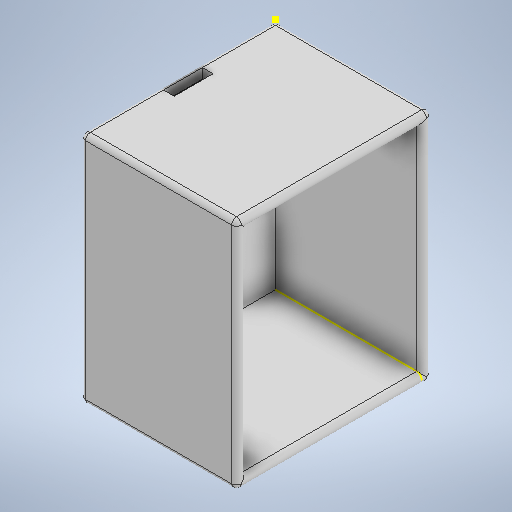
# Autodesk Inventor part: box
Saved by Autodesk Inventor 2025.2 (Build 292293000, 293)
## iProperties
Created: 2025-01-12
Part Number: box
Material: Generic
Document SubType Name: Modeling
Designer: sujay
Density: 1 g/cm^3
Appearance: Default
Author: sujay
Autodesk Inventor part; units mm, degrees
ref_plane "YZ Plane" through (0, 0, 0) normal (1, 0, 0) x (0, 1, 0)
ref_plane "XZ Plane" through (0, 0, 0) normal (0, 1, 0) x (-1, 0, 0)
ref_plane "XY Plane" through (0, 0, 0) normal (0, 0, 1) x (1, 0, 0)
sketch "Sketch1" plane through (0, 0, 0) normal (0, 0, 1) x (1, 0, 0)
  line L0 (0, 0) -> (101.6, 0)
  line L1 (101.6, 0) -> (101.6, 152.4)
  line L2 (101.6, 152.4) -> (0, 152.4)
  line L3 (0, 152.4) -> (0, 0)
  dimension "d0" = 101.6
  dimension "d1" = 152.4
  constraints: 8 end point, 2 parallel, 1 horizontal, 1 perpendicular
  measures "d0" distance of L2.end L1.end
  measures "d1" distance of L1.end L0.end
sketch "Sketch2" plane through (0, 0, 0) normal (0, 0, 1) x (1, 0, 0)
  point P0 (0, 0)
sketch "Sketch3" plane through (0, 0, 0) normal (0, 0, 1) x (1, 0, 0)
  point P0 (0, 0)
extrude "Extrusion1" add sketch "Sketch1" along normal blind 127
sketch "Sketch4" plane through (101.6, 0, 0) normal (1, 0, 0) x (0, 0, -1)
  line L0 (0, 0) -> (-127, 0) projected
  line L1 (0, 0) -> (-6.35, 0)
  line L2 (-6.35, 0) -> (-6.35, 6.35)
  line L3 (-6.35, 6.35) -> (0, 6.35)
  line L4 (0, 6.35) -> (0, 0)
  line L5 (-6.35, 6.35) -> (-120.65, 6.35)
  line L6 (-120.65, 6.35) -> (-120.65, 146.05)
  line L7 (-120.65, 146.05) -> (-6.35, 146.05)
  line L8 (-6.35, 146.05) -> (-6.35, 6.35)
  dimension "d4" = 6.35
  dimension "d5" = 6.35
  dimension "d6" = 114.3
  dimension "d7" = 139.7
  constraints: 16 end point, 4 parallel, 2 horizontal, 2 perpendicular
  measures "d4" distance of L2.end L3.end
  measures "d5" distance of L1.end L2.end
  measures "d6" distance of L6.end L7.end
  measures "d7" distance of L5.end L6.end
extrude "Extrusion2" cut sketch "Sketch4" against normal blind 95.25 contours L5 L6 L7 L8
fillet "Fillet1" radius 3.175 8 edges at (101.6, 146.05, 63.5) (101.6, 152.4, 63.5) (101.6, 76.2, 127) (101.6, 76.2, 120.65) (101.6, 76.2, 6.35) (101.6, 76.2, 0) (101.6, 6.35, 63.5) (101.6, 0, 63.5)
fillet "Fillet2" radius 3.175 8 edges at (100.6701, 151.4701, 126.0701) (49.2126, 152.4, 127) (100.6701, 151.4701, 0.9299) (49.2126, 152.4, 0) (100.6701, 0.9299, 126.0701) (49.2126, 0, 127) (100.6701, 0.9299, 0.9299) (49.2126, 0, 0)
fillet "Fillet3" radius 3.175 8 edges at (0, 0.9299, 0.9299) (0, 0, 63.5) (0, 0.9299, 126.0701) (0, 76.2, 127) (0, 151.4701, 126.0701) (0, 152.4, 63.5) (0, 151.4701, 0.9299) (0, 76.2, 0)
sketch "Sketch5" plane through (6.35, 6.35, 6.35) normal (0, 0, 1) x (1, 0, 0)
  line L0 (92.075, 0) -> (0, 0) projected
  arc A0 (95.25, -3.175) -> (92.075, 0) centre (92.075, -3.175) ccw projected
  line L1 (92.075, 0) -> (89.535, 0)
  line L2 (92.075, 0) -> (94.615, 0) construction
  line L3 (91.2996, 0) -> (88.936, -0.9299)
  point P0 (-6.35, -6.35)
  constraints: 6 end point, 2 horizontal, 1 collinear, 1 point on line
sketch "Sketch6" plane through (6.35, 6.35, 6.35) normal (0, 0, 1) x (1, 0, 0)
  point P0 (-6.35, -6.35)
sketch "Sketch7" plane through (98.425, 152.4, 123.825) normal (0, 1, 0) x (1, 0, 0)
  line L0 (-95.25, 120.65) -> (0, 120.65) projected
  line L1 (-95.25, 120.65) -> (-95.25, 73.025)
  line L2 (0, 0) -> (-95.25, 0) projected
  arc A0 (-98.425, 0) -> (-95.25, -3.175) centre (-95.25, 0) ccw projected
  line L3 (-92.075, 3.175) -> (-92.075, 117.475) projected
  line L4 (-95.25, 0) -> (-98.425, 0) projected
  line L5 (-95.25, 0) -> (-95.25, 47.625)
  line L6 (-95.25, 0) -> (-95.25, 120.65) projected
  line L7 (-95.25, 73.025) -> (-95.25, 47.625)
  line L8 (-95.25, 47.625) -> (-91.44, 47.625)
  line L9 (-91.44, 47.625) -> (-91.44, 73.025)
  line L10 (-91.44, 73.025) -> (-95.25, 73.025)
  point P0 (-98.425, 123.825)
  point P1 (-92.075, 73.025)
  point P2 (-92.075, 47.625)
  dimension "d17" = 47.625
  dimension "d20" = 47.625
  dimension "d21" = 3.81
  constraints: 12 end point, 2 parallel, 2 perpendicular, 1 collinear, 1 point on line
  measures "d17" distance of L0.start L1.end
  measures "d20" distance of L2.end L5.end
  measures "d21" distance of L8.end L5.end
sketch "Sketch8" plane through (98.425, 152.4, 123.825) normal (0, 1, 0) x (1, 0, 0)
  point P0 (-98.425, 123.825)
extrude "Extrusion3" cut sketch "Sketch7" against normal blind 6.604 contours L8 L6 L10 L3
sketch "Sketch9" plane through (98.425, 152.4, 123.825) normal (0, 1, 0) x (1, 0, 0)
  line L0 (-95.25, 73.025) -> (-92.075, 73.025) projected
  line L1 (-92.075, 73.025) -> (-92.075, 47.625) projected
  line L2 (-92.075, 73.025) -> (-92.075, 47.625)
  line L3 (-92.075, 47.625) -> (-88.265, 47.625)
  line L4 (-88.265, 47.625) -> (-88.265, 73.025)
  line L5 (-88.265, 73.025) -> (-92.075, 73.025)
  point P0 (-98.425, 123.825)
  dimension "d24" = 3.81
  constraints: 8 end point, 2 parallel, 1 perpendicular, 1 vertical
  measures "d24" distance of L3.end L1.end
extrude "Extrusion4" cut sketch "Sketch9" against normal blind 7.62
body "Solid1"
